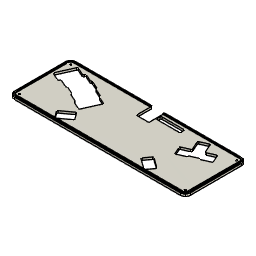
case-top v2 (Autodesk Fusion 360 design; units mm, degrees)
Autodesk Fusion 360 part; units mm, degrees
sketch "triplejump-brd" plane through (0, 0, 0) normal (0, 0, 1) x (1, 0, 0)
  line L0 (142.675, 106.5563) -> (142.925, 106.5563)
  line L1 (109.6125, 106.3063) -> (109.6125, 106.5563)
  line L2 (121.5187, 106.5563) -> (121.7687, 106.5563)
  line L3 (121.5187, 99.0562) -> (121.7687, 99.0562)
  line L4 (121.5187, 99.3062) -> (121.5187, 99.0562)
  line L5 (130.7687, 99.0562) -> (121.7687, 99.0562)
  line L6 (130.7687, 99.0562) -> (131.0187, 99.0562)
  line L7 (131.0187, 106.5563) -> (131.0187, 106.3063)
  line L8 (121.5187, 99.3062) -> (121.5187, 106.3063)
  line L9 (121.7687, 106.5563) -> (130.7687, 106.5563)
  line L10 (109.6125, 99.3062) -> (109.6125, 99.0562)
  line L11 (133.425, 99.0562) -> (133.675, 99.0562)
  line L12 (133.675, 106.5563) -> (142.675, 106.5563)
  line L13 (118.8625, 106.5563) -> (119.1125, 106.5563)
  line L14 (109.8625, 106.5563) -> (118.8625, 106.5563)
  line L15 (142.925, 99.0562) -> (142.925, 99.3062)
  line L16 (142.925, 106.3063) -> (142.925, 99.3062)
  line L17 (119.1125, 99.0562) -> (119.1125, 99.3062)
  line L18 (133.425, 106.5563) -> (133.675, 106.5563)
  line L19 (130.7687, 106.5563) -> (131.0187, 106.5563)
  line L20 (133.425, 99.3062) -> (133.425, 106.3063)
  line L21 (142.675, 99.0562) -> (142.925, 99.0562)
  line L22 (109.6125, 99.0562) -> (109.8625, 99.0562)
  spline S0 degree 3 poles (1.4645, 1.4645) (2.4021, 0.5268) (3.6739, 0) (5, 0) knots 0 0 0 0 1 1 1 1
  line L23 (133.425, 99.3062) -> (133.425, 99.0562)
  line L24 (133.425, 106.3063) -> (133.425, 106.5563)
  line L25 (142.925, 106.5563) -> (142.925, 106.3063)
  line L26 (121.5187, 106.3063) -> (121.5187, 106.5563)
  line L27 (118.8625, 99.0562) -> (109.8625, 99.0562)
  line L28 (119.1125, 106.5563) -> (119.1125, 106.3063)
  line L29 (142.675, 99.0562) -> (133.675, 99.0562)
  line L30 (119.1125, 106.3063) -> (119.1125, 99.3062)
  line L31 (118.8625, 99.0562) -> (119.1125, 99.0562)
  line L32 (109.6125, 106.5563) -> (109.8625, 106.5563)
  spline S1 degree 3 poles (335, 0) (336.3261, 0) (337.5979, 0.5268) (338.5355, 1.4645) knots 0 0 0 0 1 1 1 1
  line L33 (177, 112) -> (176.5, 112)
  line L34 (129.7687, 102.0563) -> (129.7687, 103.5563)
  line L35 (289.3678, 84.0164) -> (288.4543, 83.6096)
  line L36 (276.5782, 78.322) -> (276.1714, 79.2356)
  line L37 (110.8625, 103.5563) -> (110.8625, 102.0563)
  line L38 (271.7974, 91.5184) -> (270.8839, 91.1117)
  line L39 (54.537, 92.7011) -> (54.9437, 93.6146)
  line L40 (117.8625, 102.0563) -> (117.8625, 103.5563)
  line L41 (134.675, 103.5563) -> (134.675, 102.0563)
  line L42 (122.7687, 103.5563) -> (122.7687, 102.0563)
  spline S2 degree 3 poles (5, 112) (3.6739, 112) (2.4021, 111.4732) (1.4645, 110.5355) knots 0 0 0 0 1 1 1 1
  line L43 (131.0187, 99.0562) -> (131.0187, 99.3062)
  spline S3 degree 3 poles (0, 5) (0, 3.6739) (0.5268, 2.4021) (1.4645, 1.4645) knots 0 0 0 0 1 1 1 1
  line L44 (131.0187, 106.3063) -> (131.0187, 99.3062)
  line L45 (335, 112) -> (177, 112)
  spline S4 degree 3 poles (1.4645, 110.5355) (0.5268, 109.5979) (0, 108.3261) (0, 107) knots 0 0 0 0 1 1 1 1
  spline S5 degree 3 poles (338.5355, 1.4645) (339.4732, 2.4021) (340, 3.6739) (340, 5) knots 0 0 0 0 1 1 1 1
  line L46 (5, 0) -> (335, 0)
  line L47 (163, 112) -> (5, 112)
  line L48 (340, 5) -> (340, 107)
  spline S6 degree 3 poles (340, 107) (340, 108.3261) (339.4732, 109.5979) (338.5355, 110.5355) knots 0 0 0 0 1 1 1 1
  line L49 (0, 107) -> (0, 5)
  line L50 (163.5, 112) -> (163, 112)
  spline S7 degree 3 poles (338.5355, 110.5355) (337.5979, 111.4732) (336.3261, 112) (335, 112) knots 0 0 0 0 1 1 1 1
  line L51 (54.537, 92.7011) -> (55.4505, 92.2944)
  line L52 (288.9611, 84.9299) -> (289.3678, 84.0164)
  line L53 (140.425, 106.0563) -> (135.925, 106.0563)
  line L54 (283.6735, 96.806) -> (282.76, 96.3993)
  line L55 (59.8246, 104.5772) -> (60.2313, 105.4907)
  line L56 (73.021, 99.7964) -> (72.1074, 100.2032)
  line L57 (128.5187, 106.0563) -> (124.0187, 106.0563)
  line L58 (61.1449, 105.084) -> (60.2313, 105.4907)
  line L59 (283.6735, 96.806) -> (284.0802, 95.8925)
  line L60 (67.3266, 87.0068) -> (66.4131, 87.4135)
  line L61 (276.5782, 78.322) -> (277.4917, 78.7288)
  line L62 (112.1125, 99.5562) -> (116.6125, 99.5562)
  line L63 (66.4131, 87.4135) -> (67.3266, 87.0068)
  line L64 (288.4543, 83.6096) -> (289.3678, 84.0164)
  line L65 (67.7334, 87.9203) -> (67.3266, 87.0068)
  line L66 (141.675, 102.0563) -> (141.675, 103.5563)
  line L67 (124.0187, 99.5562) -> (128.5187, 99.5562)
  line L68 (116.6125, 106.0563) -> (112.1125, 106.0563)
  line L69 (135.925, 99.5562) -> (140.425, 99.5562)
  line L70 (73.021, 99.7964) -> (72.6142, 98.8829)
  line L71 (145.3312, 106.3063) -> (145.3312, 106.5563)
  line L72 (145.5812, 106.5563) -> (154.5812, 106.5563)
  line L73 (145.3312, 99.0562) -> (145.5812, 99.0562)
  line L74 (145.3312, 99.3062) -> (145.3312, 99.0562)
  line L75 (145.3312, 106.5563) -> (145.5812, 106.5563)
  line L76 (154.5812, 99.0562) -> (145.5812, 99.0562)
  line L77 (145.3312, 99.3062) -> (145.3312, 106.3063)
  line L78 (154.8312, 106.5563) -> (154.8312, 106.3063)
  line L79 (154.8312, 99.0562) -> (154.8312, 99.3062)
  line L80 (154.5812, 106.5563) -> (154.8312, 106.5563)
  line L81 (154.5812, 99.0562) -> (154.8312, 99.0562)
  line L82 (297.1161, 66.6133) -> (296.2026, 66.2066)
  line L83 (254.3169, 5.0503) -> (253.5079, 5.6381)
  line L84 (291.4218, 79.403) -> (290.5083, 78.9962)
  line L85 (88.7804, 24.6055) -> (87.9714, 24.0177)
  line L86 (88.7804, 24.6055) -> (89.3682, 23.7965)
  line L87 (85.6831, 5.0503) -> (86.4921, 5.6381)
  line L88 (254.8305, 80.332) -> (254.4237, 81.2455)
  line L89 (96.2004, 12.6915) -> (97.0094, 13.2793)
  line L90 (284.3265, 60.919) -> (285.2401, 61.3257)
  line L91 (260.118, 68.4559) -> (259.7113, 69.3694)
  line L92 (85.6831, 5.0503) -> (85.0953, 5.8593)
  line L93 (242.9906, 13.2793) -> (243.7996, 12.6915)
  line L94 (246.1187, 53.0628) -> (245.7119, 53.9763)
  line L95 (258.5016, 59.6706) -> (258.9083, 58.7571)
  line L96 (41.1761, 75.1935) -> (40.2625, 75.6002)
  line L97 (294.9241, 83.9526) -> (294.5174, 84.8661)
  line L98 (68.4801, 77.2672) -> (68.8868, 78.1808)
  line L99 (302.6725, 66.5495) -> (303.586, 66.9562)
  line L100 (296.2026, 66.2066) -> (297.1161, 66.6133)
  line L101 (254.9047, 5.8593) -> (254.3169, 5.0503)
  line L102 (267.2134, 86.9398) -> (267.6201, 86.0263)
  line L103 (326.5959, 94.0731) -> (327.0026, 93.1595)
  line L104 (63.1925, 65.3911) -> (63.5993, 66.3047)
  line L105 (297.8917, 79.7459) -> (296.9782, 79.3391)
  line L106 (250.6318, 23.7965) -> (251.2196, 24.6055)
  line L107 (267.2134, 86.9398) -> (266.2998, 86.5331)
  line L108 (253.5079, 5.6381) -> (254.3169, 5.0503)
  line L109 (296.7094, 67.5269) -> (297.1161, 66.6133)
  line L110 (262.5459, 16.3765) -> (261.9581, 15.5675)
  line L111 (279.5457, 74.1154) -> (278.6322, 73.7086)
  line L112 (260.118, 68.4559) -> (261.0316, 68.8626)
  line L113 (306.8002, 89.2401) -> (307.7138, 89.6469)
  line L114 (76.3889, 60.6104) -> (75.9822, 59.6968)
  line L115 (302.6725, 66.5495) -> (302.2657, 67.4631)
  line L116 (272.5009, 75.0637) -> (272.9077, 74.1502)
  line L117 (262.5459, 16.3765) -> (261.7368, 16.9643)
  line L118 (28.3864, 80.8878) -> (29.3, 80.4811)
  line L119 (334.751, 75.7565) -> (333.8374, 75.3498)
  line L120 (78.2632, 16.9643) -> (77.4541, 16.3765)
  line L121 (291.4218, 79.403) -> (291.8286, 78.4894)
  line L122 (242.9906, 13.2793) -> (243.5784, 14.0883)
  line L123 (75.0686, 60.1035) -> (75.9822, 59.6968)
  line L124 (321.3083, 105.9492) -> (320.3948, 105.5424)
  line L125 (251.4063, 41.1867) -> (252.3198, 41.5934)
  line L126 (252.0286, 24.0177) -> (251.2196, 24.6055)
  line L127 (333.8374, 75.3498) -> (334.751, 75.7565)
  line L128 (258.5016, 59.6706) -> (257.588, 59.2639)
  line L129 (284.3265, 60.919) -> (283.9198, 61.8326)
  line L130 (329.0567, 88.5461) -> (328.1431, 88.1394)
  line L131 (279.0389, 72.7951) -> (278.6322, 73.7086)
  line L132 (255.3373, 81.6523) -> (254.4237, 81.2455)
  line L133 (81.6765, 72.4864) -> (81.2697, 71.5729)
  line L134 (272.9077, 74.1502) -> (271.9941, 73.7435)
  line L135 (271.9941, 73.7435) -> (272.9077, 74.1502)
  line L136 (78.0419, 15.5675) -> (77.4541, 16.3765)
  line L137 (327.0026, 93.1595) -> (326.0891, 92.7528)
  line L138 (147.8312, 99.5562) -> (152.3312, 99.5562)
  line L139 (256.4476, 64.284) -> (255.534, 63.8773)
  line L140 (294.9241, 83.9526) -> (295.8377, 84.3593)
  line L141 (28.3864, 80.8878) -> (28.7932, 81.8013)
  line L142 (75.9822, 59.6968) -> (75.0686, 60.1035)
  line L143 (271.2906, 90.1981) -> (270.8839, 91.1117)
  line L144 (53.3659, 87.6977) -> (52.4523, 88.1045)
  line L145 (153.5812, 102.0563) -> (153.5812, 103.5563)
  line L146 (46.8704, 87.9831) -> (45.9568, 88.3899)
  line L147 (58.6341, 70.0273) -> (59.5477, 69.6205)
  line L148 (302.0195, 102.4365) -> (302.4262, 101.523)
  line L149 (40.2625, 75.6002) -> (41.1761, 75.1935)
  line L150 (96.4216, 14.0883) -> (97.0094, 13.2793)
  line L151 (316.6738, 81.9383) -> (316.267, 82.8518)
  line L152 (263.7892, 47.7945) -> (264.1959, 46.881)
  line L153 (326.0891, 92.7528) -> (327.0026, 93.1595)
  line L154 (52.0456, 87.1909) -> (52.4523, 88.1045)
  line L155 (81.6765, 72.4864) -> (80.7629, 72.8932)
  line L156 (309.7678, 85.0335) -> (308.8542, 84.6267)
  line L157 (263.2823, 46.4743) -> (264.1959, 46.881)
  line L158 (309.4322, 100.6616) -> (308.5187, 100.2549)
  line L159 (314.5486, 71.8371) -> (315.4621, 72.2438)
  line L160 (309.7678, 85.0335) -> (310.1745, 84.1199)
  line L161 (264.1959, 46.881) -> (263.2823, 46.4743)
  line L162 (321.9613, 70.0622) -> (322.8749, 70.4689)
  line L163 (34.9943, 93.2707) -> (34.0808, 93.6774)
  line L164 (302.0195, 102.4365) -> (301.1059, 102.0298)
  line L165 (307.7138, 89.6469) -> (306.8002, 89.2401)
  line L166 (46.8704, 87.9831) -> (46.4637, 87.0696)
  line L167 (297.3849, 78.4256) -> (296.9782, 79.3391)
  line L168 (290.1434, 97.1489) -> (289.2298, 96.7422)
  line L169 (33.674, 92.7639) -> (34.0808, 93.6774)
  line L170 (307.307, 90.5604) -> (307.7138, 89.6469)
  line L171 (314.213, 87.4652) -> (313.8063, 88.3788)
  line L172 (246.6255, 54.3831) -> (245.7119, 53.9763)
  line L173 (315.0554, 73.1574) -> (315.4621, 72.2438)
  line L174 (69.8004, 77.774) -> (68.8868, 78.1808)
  line L175 (251.4063, 41.1867) -> (250.9995, 42.1002)
  line L176 (46.758, 75.3148) -> (47.6716, 74.9081)
  line L177 (97.0094, 13.2793) -> (96.2004, 12.6915)
  line L178 (321.9613, 70.0622) -> (321.5546, 70.9757)
  line L179 (41.5828, 76.107) -> (41.1761, 75.1935)
  line L180 (238.8772, 71.7861) -> (237.9636, 71.3794)
  line L181 (280.656, 56.7472) -> (279.7425, 56.3404)
  line L182 (267.8664, 51.0528) -> (267.4596, 51.9664)
  line L183 (314.213, 87.4652) -> (315.1266, 87.872)
  line L184 (238.3703, 70.4658) -> (237.9636, 71.3794)
  line L185 (317.1806, 83.2586) -> (316.267, 82.8518)
  line L186 (263.0856, 64.2492) -> (262.1721, 63.8425)
  line L187 (334.3442, 76.67) -> (334.751, 75.7565)
  line L188 (274.9617, 69.5368) -> (275.3684, 68.6232)
  line L189 (315.4621, 72.2438) -> (314.5486, 71.8371)
  line L190 (267.8664, 51.0528) -> (268.7799, 51.4596)
  line L191 (329.0567, 88.5461) -> (329.4634, 87.6326)
  line L192 (63.1925, 65.3911) -> (64.1061, 64.9844)
  line L193 (255.534, 63.8773) -> (256.4476, 64.284)
  line L194 (250.7532, 77.0737) -> (251.16, 76.1601)
  line L195 (289.6366, 95.8286) -> (289.2298, 96.7422)
  line L196 (243.6579, 58.5897) -> (243.2512, 59.5033)
  line L197 (308.9254, 99.3413) -> (308.5187, 100.2549)
  line L198 (280.2493, 57.6607) -> (280.656, 56.7472)
  line L199 (321.3083, 105.9492) -> (321.7151, 105.0356)
  line L200 (250.7532, 77.0737) -> (249.8397, 76.6669)
  line L201 (65.242, 82.4102) -> (64.3284, 82.8169)
  line L202 (59.5477, 69.6205) -> (58.6341, 70.0273)
  line L203 (274.9617, 69.5368) -> (274.0482, 69.1301)
  line L204 (243.6579, 58.5897) -> (244.5715, 58.9965)
  line L205 (146.5812, 103.5563) -> (146.5812, 102.0563)
  line L206 (59.9544, 70.5341) -> (59.5477, 69.6205)
  line L207 (65.242, 82.4102) -> (64.8352, 81.4966)
  line L208 (46.758, 75.3148) -> (47.1648, 76.2284)
  line L209 (279.7425, 56.3404) -> (280.656, 56.7472)
  line L210 (152.3312, 106.0563) -> (147.8312, 106.0563)
  line L211 (262.5788, 62.9289) -> (262.1721, 63.8425)
  line L212 (256.0408, 65.1976) -> (256.4476, 64.284)
  circle A0 centre (5, 107) radius 1.6
  circle A1 centre (5, 5) radius 1.6
  circle A2 centre (335, 107) radius 1.6
  circle A3 centre (335, 5) radius 1.6
  spline S8 degree 3 poles (339.2426, 0.7574) (340.3676, 1.8823) (341, 3.4091) (341, 5) knots 0 0 0 0 1 1 1 1
  line L213 (341, 5) -> (341, 107)
  spline S9 degree 3 poles (341, 107) (341, 108.5909) (340.3676, 110.1177) (339.2426, 111.2426) knots 0 0 0 0 1 1 1 1
  spline S10 degree 3 poles (339.2426, 111.2426) (338.1177, 112.3676) (336.5909, 113) (335, 113) knots 0 0 0 0 1 1 1 1
  line L214 (335, 113) -> (177, 113)
  line L215 (177, 113) -> (5, 113)
  spline S11 degree 3 poles (5, 113) (3.4091, 113) (1.8823, 112.3676) (0.7574, 111.2426) knots 0 0 0 0 1 1 1 1
  spline S12 degree 3 poles (0.7574, 111.2426) (-0.3676, 110.1177) (-1, 108.5909) (-1, 107) knots 0 0 0 0 1 1 1 1
  line L216 (-1, 107) -> (-1, 5)
  spline S13 degree 3 poles (-1, 5) (-1, 3.4091) (-0.3676, 1.8823) (0.7574, 0.7574) knots 0 0 0 0 1 1 1 1
  spline S14 degree 3 poles (0.7574, 0.7574) (1.8823, -0.3676) (3.4091, -1) (5, -1) knots 0 0 0 0 1 1 1 1
  line L217 (5, -1) -> (335, -1)
  spline S15 degree 3 poles (335, -1) (336.5909, -1) (338.1177, -0.3676) (339.2426, 0.7574) knots 0 0 0 0 1 1 1 1
  line L218 (68.5336, 83.0202) -> (69.3276, 84.74)
  line L219 (75.6348, 98.9062) -> (69.3276, 84.74)
  line L220 (60.4613, 107.8512) -> (74.6212, 101.5468)
  line L221 (51.5191, 92.6839) -> (57.8207, 106.8376)
  line L222 (50.6964, 90.902) -> (51.5191, 92.6839)
  line L223 (34.3108, 96.038) -> (48.0671, 89.9133)
  line L224 (25.7725, 81.7779) -> (31.6702, 95.0243)
  line L225 (41.2587, 72.6938) -> (26.7862, 79.1374)
  line L226 (59.2192, 67.3038) -> (45.5688, 73.3814)
  line L227 (75.7522, 57.3363) -> (61.5922, 63.6407)
  line L228 (84.2904, 71.5963) -> (78.3927, 58.3499)
  line L229 (69.5359, 80.3547) -> (83.2768, 74.2369)
  line L230 (235.3496, 70.4892) -> (248.9957, 39.8398)
  line L231 (251.6363, 38.8261) -> (265.7962, 45.1306)
  line L232 (282.2563, 54.9968) -> (268.1688, 48.7246)
  line L233 (298.3054, 64.6799) -> (284.6289, 58.5908)
  line L234 (302.5639, 64.0382) -> (316.6513, 70.3103)
  line L235 (319.2919, 69.2967) -> (319.5508, 68.7153)
  line L236 (336.3513, 74.0061) -> (322.1913, 67.7016)
  line L237 (337.3649, 76.6466) -> (323.7189, 107.2961)
  line L238 (321.0783, 108.3097) -> (307.3295, 102.1883)
  line L239 (304.6889, 103.202) -> (304.43, 103.7834)
  line L240 (288.0406, 98.6757) -> (301.7895, 104.7971)
  line L241 (268.9449, 92.7114) -> (283.7822, 99.3173)
  line L242 (266.5723, 89.1173) -> (252.4847, 82.8451)
  line L243 (250.1121, 79.2512) -> (236.3633, 73.1298)
  line L244 (154.8312, 99.0562) -> (154.8312, 106.5563)
  line L245 (109.6125, 99.0562) -> (109.6125, 106.5563)
  line L246 (153.8312, 98.0562) -> (110.6125, 98.0562)
  line L247 (108.6125, 100.0562) -> (108.6125, 105.5563)
  line L248 (110.6125, 107.5563) -> (153.8312, 107.5563)
  line L249 (155.8312, 105.5563) -> (155.8312, 100.0562)
  line L250 (102.5792, 14.5449) -> (82.7583, 0.1441)
  line L251 (79.9647, 0.5866) -> (71.4418, 12.3173)
  line L252 (71.8843, 15.1109) -> (91.7052, 29.5117)
  line L253 (94.4988, 29.0692) -> (103.0217, 17.3385)
  line L254 (257.2417, 0.1441) -> (237.4208, 14.5449)
  line L255 (236.9783, 17.3385) -> (245.5012, 29.0692)
  line L256 (248.2948, 29.5117) -> (268.1157, 15.1109)
  line L257 (268.5582, 12.3173) -> (260.0353, 0.5866)
  arc A4 (60.4613, 107.8512) -> (57.8207, 106.8376) centre (59.6478, 106.0241) ccw
  arc A5 (75.6348, 98.9062) -> (74.6212, 101.5468) centre (73.8077, 99.7197) ccw
  arc A6 (68.5336, 83.0202) -> (69.5359, 80.3547) centre (70.3494, 82.1818) ccw
  arc A7 (84.2904, 71.5963) -> (83.2768, 74.2369) centre (82.4633, 72.4098) ccw
  arc A8 (75.7522, 57.3363) -> (78.3927, 58.3499) centre (76.5656, 59.1634) ccw
  arc A9 (60.4057, 65.4723) -> (61.5922, 63.6407) centre (62.4057, 65.4678) ccw
  arc A10 (60.4057, 65.4723) -> (59.2192, 67.3038) centre (58.4057, 65.4768) ccw
  arc A11 (45.5688, 73.3814) -> (43.4138, 73.0376) centre (44.7554, 71.5543) ccw
  arc A12 (41.2587, 72.6938) -> (43.4138, 73.0376) centre (42.0722, 74.5209) ccw
  arc A13 (25.7725, 81.7779) -> (26.7862, 79.1374) centre (27.5996, 80.9645) ccw
  arc A14 (34.3108, 96.038) -> (31.6702, 95.0243) centre (33.4973, 94.2109) ccw
  arc A15 (48.0671, 89.9133) -> (50.6964, 90.902) centre (48.8806, 91.7403) ccw
  arc A16 (94.4988, 29.0692) -> (91.7052, 29.5117) centre (92.8808, 27.8936) ccw
  arc A17 (102.5792, 14.5449) -> (103.0217, 17.3385) centre (101.4037, 16.1629) ccw
  arc A18 (79.9647, 0.5866) -> (82.7583, 0.1441) centre (81.5827, 1.7622) ccw
  arc A19 (71.8843, 15.1109) -> (71.4418, 12.3173) centre (73.0598, 13.4929) ccw
  arc A20 (248.2948, 29.5117) -> (245.5012, 29.0692) centre (247.1192, 27.8936) ccw
  arc A21 (268.5582, 12.3173) -> (268.1157, 15.1109) centre (266.9402, 13.4929) ccw
  arc A22 (257.2417, 0.1441) -> (260.0353, 0.5866) centre (258.4173, 1.7622) ccw
  arc A23 (236.9783, 17.3385) -> (237.4208, 14.5449) centre (238.5963, 16.1629) ccw
  arc A24 (236.3633, 73.1298) -> (235.3496, 70.4892) centre (237.1767, 71.3027) ccw
  arc A25 (248.9957, 39.8398) -> (251.6363, 38.8261) centre (250.8228, 40.6532) ccw
  arc A26 (265.7962, 45.1306) -> (266.9825, 46.9276) centre (264.9828, 46.9577) ccw
  arc A27 (268.1688, 48.7246) -> (266.9825, 46.9276) centre (268.9823, 46.8975) ccw
  arc A28 (282.2563, 54.9968) -> (283.4426, 56.7938) centre (281.4429, 56.8239) ccw
  arc A29 (284.6289, 58.5908) -> (283.4426, 56.7938) centre (285.4424, 56.7637) ccw
  arc A30 (300.4346, 64.359) -> (298.3054, 64.6799) centre (299.1188, 62.8528) ccw
  arc A31 (300.4346, 64.359) -> (302.5639, 64.0382) centre (301.7504, 65.8653) ccw
  arc A32 (319.2919, 69.2967) -> (316.6513, 70.3103) centre (317.4648, 68.4832) ccw
  arc A33 (319.5508, 68.7153) -> (322.1913, 67.7016) centre (321.3779, 69.5287) ccw
  arc A34 (336.3513, 74.0061) -> (337.3649, 76.6466) centre (335.5378, 75.8332) ccw
  arc A35 (323.7189, 107.2961) -> (321.0783, 108.3097) centre (321.8918, 106.4826) ccw
  arc A36 (304.6889, 103.202) -> (307.3295, 102.1883) centre (306.516, 104.0154) ccw
  arc A37 (304.43, 103.7834) -> (301.7895, 104.7971) centre (302.6029, 102.97) ccw
  arc A38 (285.9114, 98.9965) -> (288.0406, 98.6757) centre (287.2271, 100.5028) ccw
  arc A39 (285.9114, 98.9965) -> (283.7822, 99.3173) centre (284.5956, 97.4902) ccw
  arc A40 (266.5723, 89.1173) -> (267.7586, 90.9143) centre (265.7588, 90.9444) ccw
  arc A41 (268.9449, 92.7114) -> (267.7586, 90.9143) centre (269.7584, 90.8843) ccw
  arc A42 (250.1121, 79.2512) -> (251.2984, 81.0482) centre (249.2987, 81.0783) ccw
  arc A43 (252.4847, 82.8451) -> (251.2984, 81.0482) centre (253.2982, 81.0181) ccw
  line L258 (179, 112) -> (161, 112)
  line L259 (161, 112) -> (161, 88.5)
  line L260 (161, 88.5) -> (179, 88.5)
  line L261 (179, 88.5) -> (179, 112)
  line L262 (333.4123, 7.75) -> (331.8246, 5)
  line L263 (331.8246, 5) -> (333.4123, 2.25)
  line L264 (333.4123, 2.25) -> (336.5877, 2.25)
  line L265 (336.5877, 2.25) -> (338.1754, 5)
  line L266 (338.1754, 5) -> (336.5877, 7.75)
  line L267 (336.5877, 7.75) -> (333.4123, 7.75)
  line L268 (3.4123, 109.75) -> (1.8246, 107)
  line L269 (1.8246, 107) -> (3.4123, 104.25)
  line L270 (3.4123, 104.25) -> (6.5877, 104.25)
  line L271 (6.5877, 104.25) -> (8.1754, 107)
  line L272 (8.1754, 107) -> (6.5877, 109.75)
  line L273 (6.5877, 109.75) -> (3.4123, 109.75)
  line L274 (6.5877, 7.75) -> (3.4123, 7.75)
  line L275 (8.1754, 5) -> (6.5877, 7.75)
  line L276 (3.4123, 7.75) -> (1.8246, 5)
  line L277 (1.8246, 5) -> (3.4123, 2.25)
  line L278 (6.5877, 2.25) -> (8.1754, 5)
  line L279 (3.4123, 2.25) -> (6.5877, 2.25)
  line L280 (333.4123, 109.75) -> (331.8246, 107)
  line L281 (336.5877, 109.75) -> (333.4123, 109.75)
  line L282 (338.1754, 107) -> (336.5877, 109.75)
  line L283 (331.8246, 107) -> (333.4123, 104.25)
  line L284 (333.4123, 104.25) -> (336.5877, 104.25)
  line L285 (336.5877, 104.25) -> (338.1754, 107)
  arc A44 (77.9187, 97.8894) -> (75.6381, 103.8307) centre (73.8077, 99.7197) ccw
  line L286 (61.4781, 110.1351) -> (75.6381, 103.8307)
  arc A45 (61.4781, 110.1351) -> (55.5368, 107.8544) centre (59.6478, 106.0241) ccw
  line L287 (49.2421, 93.7163) -> (55.5368, 107.8544)
  line L288 (48.6333, 92.3977) -> (49.2421, 93.7163)
  line L289 (35.3276, 98.3218) -> (48.6333, 92.3977)
  arc A46 (35.3276, 98.3218) -> (29.3864, 96.0412) centre (33.4973, 94.2109) ccw
  line L290 (23.4887, 82.7948) -> (29.3864, 96.0412)
  arc A47 (23.4887, 82.7948) -> (25.7693, 76.8535) centre (27.5996, 80.9645) ccw
  line L291 (40.2419, 70.4099) -> (25.7693, 76.8535)
  arc A48 (40.2419, 70.4099) -> (44.8372, 70.9705) centre (42.0722, 74.5209) ccw
  line L292 (57.9171, 65.147) -> (44.8372, 70.9705)
  arc A49 (57.9171, 65.147) -> (60.5754, 61.3568) centre (62.4057, 65.4678) ccw
  line L293 (74.7353, 55.0524) -> (60.5754, 61.3568)
  arc A50 (74.7353, 55.0524) -> (80.6766, 57.3331) centre (76.5656, 59.1634) ccw
  line L294 (86.5743, 70.5795) -> (80.6766, 57.3331)
  arc A51 (86.5743, 70.5795) -> (84.2936, 76.5208) centre (82.4633, 72.4098) ccw
  line L295 (71.0158, 82.4324) -> (84.2936, 76.5208)
  line L296 (71.0158, 82.4324) -> (71.6046, 83.7076)
  line L297 (77.9187, 97.8894) -> (71.6046, 83.7076)
  arc A52 (108.6125, 100.0562) -> (110.6125, 98.0562) centre (110.6125, 100.0562) ccw
  arc A53 (110.6125, 107.5563) -> (108.6125, 105.5563) centre (110.6125, 105.5563) ccw
  arc A54 (155.8312, 105.5563) -> (153.8312, 107.5563) centre (153.8312, 105.5563) ccw
  arc A55 (153.8312, 98.0562) -> (155.8312, 100.0562) centre (153.8312, 100.0562) ccw
  spline S16 degree 3 poles (-0.6569, -0.6569) (0.8429, -2.1566) (2.8791, -3) (5, -3) knots 0 0 0 0 1 1 1 1
  line L298 (5, -3) -> (335, -3)
  spline S17 degree 3 poles (335, -3) (337.1209, -3) (339.1571, -2.1566) (340.6569, -0.6569) knots 0 0 0 0 1 1 1 1
  spline S18 degree 3 poles (340.6569, -0.6569) (342.1566, 0.8429) (343, 2.8791) (343, 5) knots 0 0 0 0 1 1 1 1
  line L299 (343, 5) -> (343, 107)
  spline S19 degree 3 poles (343, 107) (343, 109.1209) (342.1566, 111.1571) (340.6569, 112.6569) knots 0 0 0 0 1 1 1 1
  spline S20 degree 3 poles (340.6569, 112.6569) (339.1571, 114.1566) (337.1209, 115) (335, 115) knots 0 0 0 0 1 1 1 1
  line L300 (335, 115) -> (177, 115)
  line L301 (177, 115) -> (5, 115)
  spline S21 degree 3 poles (5, 115) (2.8791, 115) (0.8429, 114.1566) (-0.6569, 112.6569) knots 0 0 0 0 1 1 1 1
  spline S22 degree 3 poles (-0.6569, 112.6569) (-2.1566, 111.1571) (-3, 109.1209) (-3, 107) knots 0 0 0 0 1 1 1 1
  line L302 (-3, 107) -> (-3, 5)
  spline S23 degree 3 poles (-3, 5) (-3, 2.8791) (-2.1566, 0.8429) (-0.6569, -0.6569) knots 0 0 0 0 1 1 1 1
  spline S24 degree 3 poles (342.0711, 114.0711) (340.1966, 115.9456) (337.651, 117) (335, 117) knots 0 0 0 0 1 1 1 1
  line L303 (335, 117) -> (177, 117)
  line L304 (177, 117) -> (5, 117)
  spline S25 degree 3 poles (5, 117) (2.349, 117) (-0.1966, 115.9456) (-2.0711, 114.0711) knots 0 0 0 0 1 1 1 1
  spline S26 degree 3 poles (-2.0711, 114.0711) (-3.9456, 112.1966) (-5, 109.651) (-5, 107) knots 0 0 0 0 1 1 1 1
  line L305 (-5, 107) -> (-5, 5)
  spline S27 degree 3 poles (-5, 5) (-5, 2.349) (-3.9456, -0.1966) (-2.0711, -2.0711) knots 0 0 0 0 1 1 1 1
  spline S28 degree 3 poles (-2.0711, -2.0711) (-0.1966, -3.9456) (2.349, -5) (5, -5) knots 0 0 0 0 1 1 1 1
  line L306 (5, -5) -> (335, -5)
  spline S29 degree 3 poles (335, -5) (337.651, -5) (340.1966, -3.9456) (342.0711, -2.0711) knots 0 0 0 0 1 1 1 1
  spline S30 degree 3 poles (342.0711, -2.0711) (343.9456, -0.1966) (345, 2.349) (345, 5) knots 0 0 0 0 1 1 1 1
  line L307 (345, 5) -> (345, 107)
  spline S31 degree 3 poles (345, 107) (345, 109.651) (343.9456, 112.1966) (342.0711, 114.0711) knots 0 0 0 0 1 1 1 1
  arc A56 (158.3312, 105.5563) -> (153.8312, 110.0563) centre (153.8312, 105.5563) ccw
  line L308 (110.6125, 110.0563) -> (153.8312, 110.0563)
  arc A57 (110.6125, 110.0563) -> (106.1125, 105.5563) centre (110.6125, 105.5563) ccw
  line L309 (106.1125, 100.0562) -> (106.1125, 105.5563)
  arc A58 (106.1125, 100.0562) -> (110.6125, 95.5562) centre (110.6125, 100.0562) ccw
  line L310 (153.8312, 95.5562) -> (110.6125, 95.5562)
  arc A59 (153.8312, 95.5562) -> (158.3312, 100.0562) centre (153.8312, 100.0562) ccw
  line L311 (158.3312, 105.5563) -> (158.3312, 100.0562)
  arc A60 (96.5213, 30.5387) -> (90.2357, 31.5342) centre (92.8808, 27.8936) ccw
  line L312 (70.4148, 17.1335) -> (90.2357, 31.5342)
  arc A61 (70.4148, 17.1335) -> (69.4193, 10.8479) centre (73.0598, 13.4929) ccw
  line L313 (77.9422, -0.8829) -> (69.4193, 10.8479)
  arc A62 (77.9422, -0.8829) -> (84.2278, -1.8784) centre (81.5827, 1.7622) ccw
  line L314 (104.0487, 12.5223) -> (84.2278, -1.8784)
  arc A63 (104.0487, 12.5223) -> (105.0442, 18.8079) centre (101.4037, 16.1629) ccw
  line L315 (96.5213, 30.5387) -> (105.0442, 18.8079)
  arc A64 (270.5807, 10.8479) -> (269.5852, 17.1335) centre (266.9402, 13.4929) ccw
  line L316 (249.7643, 31.5342) -> (269.5852, 17.1335)
  arc A65 (249.7643, 31.5342) -> (243.4787, 30.5387) centre (247.1192, 27.8936) ccw
  line L317 (234.9558, 18.8079) -> (243.4787, 30.5387)
  arc A66 (234.9558, 18.8079) -> (235.9513, 12.5223) centre (238.5963, 16.1629) ccw
  line L318 (255.7722, -1.8784) -> (235.9513, 12.5223)
  arc A67 (255.7722, -1.8784) -> (262.0578, -0.8829) centre (258.4173, 1.7622) ccw
  line L319 (270.5807, 10.8479) -> (262.0578, -0.8829)
  arc A68 (283.2732, 52.7129) -> (285.9257, 56.4315) centre (281.4429, 56.8239) ccw
  line L320 (299.0422, 62.2714) -> (285.9257, 56.4315)
  arc A69 (299.0422, 62.2714) -> (303.5807, 61.7543) centre (301.7504, 65.8653) ccw
  line L321 (303.5807, 61.7543) -> (317.2114, 67.8231)
  line L322 (317.2114, 67.8231) -> (317.2669, 67.6984)
  arc A70 (317.2669, 67.6984) -> (323.2082, 65.4178) centre (321.3779, 69.5287) ccw
  line L323 (337.3681, 71.7222) -> (323.2082, 65.4178)
  arc A71 (337.3681, 71.7222) -> (339.6488, 77.6635) centre (335.5378, 75.8332) ccw
  line L324 (339.6488, 77.6635) -> (326.0027, 108.3129)
  arc A72 (326.0027, 108.3129) -> (320.0615, 110.5936) centre (321.8918, 106.4826) ccw
  line L325 (320.0615, 110.5936) -> (306.7694, 104.6756)
  line L326 (306.7694, 104.6756) -> (306.7139, 104.8003)
  arc A73 (306.7139, 104.8003) -> (300.7726, 107.0809) centre (302.6029, 102.97) ccw
  line L327 (287.3037, 101.0842) -> (300.7726, 107.0809)
  arc A74 (287.3037, 101.0842) -> (282.7653, 101.6012) centre (284.5956, 97.4902) ccw
  line L328 (267.9281, 94.9952) -> (282.7653, 101.6012)
  arc A75 (267.9281, 94.9952) -> (265.2755, 91.2766) centre (269.7584, 90.8843) ccw
  line L329 (265.2755, 91.2766) -> (251.4679, 85.129)
  arc A76 (251.4679, 85.129) -> (248.8153, 81.4104) centre (253.2982, 81.0181) ccw
  line L330 (248.8153, 81.4104) -> (235.3464, 75.4137)
  arc A77 (235.3464, 75.4137) -> (233.0658, 69.4724) centre (237.1767, 71.3027) ccw
  line L331 (233.0658, 69.4724) -> (246.7119, 38.8229)
  arc A78 (246.7119, 38.8229) -> (252.6531, 36.5423) centre (250.8228, 40.6532) ccw
  line L332 (252.6531, 36.5423) -> (266.8131, 42.8467)
  arc A79 (266.8131, 42.8467) -> (269.4656, 46.5654) centre (264.9828, 46.9577) ccw
  line L333 (283.2732, 52.7129) -> (269.4656, 46.5654)
  line L334 (161, 112) -> (179, 112)
  line L335 (179, 112) -> (179, 117)
  line L336 (179, 117) -> (161, 117)
  line L337 (161, 117) -> (161, 112)
  line L338 (161, 117) -> (161, 88.5)
  line L339 (179, 88.5) -> (179, 117)
  line L340 (157.5, 115) -> (157.5, 87)
  line L341 (159.5, 85) -> (180.5, 85)
  line L342 (182.5, 87) -> (182.5, 115)
  line L343 (5, 117) -> (155.5, 117)
  line L344 (184.5, 117) -> (335, 117)
  arc A80 (157.5, 87) -> (159.5, 85) centre (159.5, 87) ccw
  arc A81 (180.5, 85) -> (182.5, 87) centre (180.5, 87) ccw
  arc A82 (184.5, 117) -> (182.5, 115) centre (184.5, 115) ccw
  arc A83 (157.5, 115) -> (155.5, 117) centre (155.5, 115) ccw
  circle A84 centre (5, 107) radius 3
  circle A85 centre (5, 5) radius 3
  circle A86 centre (335, 5) radius 3
  circle A87 centre (335, 107) radius 3
  point P0 (335, 5)
  point P1 (335, 5)
  dimension "d25" = 2
  dimension "d28" = -2.5
  dimension "d29" = 2
  dimension "d30" = 2
  dimension "d31" = 2
  dimension "d32" = 2
  dimension "d33" = 4
  dimension "d34" = -2.5
  dimension "d35" = -2.5
  dimension "d36" = -2.5
  dimension "d37" = -2.5
  dimension "d60" = 2
  dimension "d61" = 2
  dimension "d62" = 2
  dimension "d63" = 2
  constraint perpendicular L80 L244
  constraint perpendicular L32 L245
  constraint tangent L220 A4
  constraint tangent L221 A4
  constraint tangent L219 A5
  constraint tangent L220 A5
  constraint equal A4 A5
  constraint tangent L218 A6
  constraint tangent L229 A6
  constraint equal A4 A6
  constraint tangent L229 A7
  constraint tangent L228 A7
  constraint equal A4 A7
  constraint tangent L228 A8
  constraint tangent L227 A8
  constraint equal A4 A8
  constraint tangent L227 A9
  constraint equal A4 A9
  constraint tangent L226 A10
  constraint tangent A9 A10
  constraint equal A4 A10
  constraint tangent L226 A11
  constraint equal A4 A11
  constraint tangent L225 A12
  constraint tangent A11 A12
  constraint equal A4 A12
  constraint tangent L225 A13
  constraint tangent L224 A13
  constraint equal A4 A13
  constraint tangent L224 A14
  constraint tangent L223 A14
  constraint equal A4 A14
  constraint tangent L223 A15
  constraint tangent L222 A15
  constraint equal A4 A15
  constraint tangent L252 A16
  constraint tangent L253 A16
  constraint equal A4 A16
  constraint tangent L253 A17
  constraint tangent L250 A17
  constraint equal A4 A17
  constraint tangent L250 A18
  constraint tangent L251 A18
  constraint equal A4 A18
  constraint tangent L251 A19
  constraint tangent L252 A19
  constraint equal A4 A19
  constraint tangent L255 A20
  constraint tangent L256 A20
  constraint equal A4 A20
  constraint tangent L257 A21
  constraint tangent L256 A21
  constraint equal A4 A21
  constraint tangent L257 A22
  constraint tangent L254 A22
  constraint equal A4 A22
  constraint tangent L254 A23
  constraint tangent L255 A23
  constraint equal A4 A23
  constraint tangent L243 A24
  constraint tangent L230 A24
  constraint equal A4 A24
  constraint tangent L230 A25
  constraint tangent L231 A25
  constraint equal A4 A25
  constraint tangent L231 A26
  constraint equal A4 A26
  constraint tangent L232 A27
  constraint tangent A26 A27
  constraint equal A4 A27
  constraint tangent L232 A28
  constraint equal A4 A28
  constraint tangent L233 A29
  constraint tangent A28 A29
  constraint equal A4 A29
  constraint tangent L233 A30
  constraint equal A4 A30
  constraint tangent L234 A31
  constraint tangent A30 A31
  constraint equal A4 A31
  constraint tangent L234 A32
  constraint tangent L235 A32
  constraint equal A4 A32
  constraint tangent L235 A33
  constraint tangent L236 A33
  constraint equal A4 A33
  constraint tangent L236 A34
  constraint tangent L237 A34
  constraint equal A4 A34
  constraint tangent L237 A35
  constraint tangent L238 A35
  constraint equal A4 A35
  constraint tangent L238 A36
  constraint tangent L239 A36
  constraint equal A4 A36
  constraint tangent L239 A37
  constraint tangent L240 A37
  constraint equal A4 A37
  constraint tangent L240 A38
  constraint equal A4 A38
  constraint tangent L241 A39
  constraint tangent A38 A39
  constraint equal A4 A39
  constraint tangent L242 A40
  constraint equal A4 A40
  constraint tangent L241 A41
  constraint tangent A40 A41
  constraint equal A4 A41
  constraint tangent L243 A42
  constraint equal A4 A42
  constraint tangent L242 A43
  constraint tangent A42 A43
  constraint equal A4 A43
  constraint horizontal L258
  constraint vertical L259
  constraint horizontal L260
  constraint vertical L261
  constraint coincident P1 P0
  constraint tangent L246 A52
  constraint tangent L248 A53
  constraint tangent L247 A53
  constraint tangent L248 A54
  constraint tangent L249 A54
  constraint equal A53 A54
  constraint tangent L249 A55
  constraint tangent L246 A55
  constraint horizontal L334
  constraint vertical L335
  constraint horizontal L336
  constraint vertical L337
  constraint coincident L303 L335.end
  constraint perpendicular L336 L339
  constraint tangent L340 A80
  constraint tangent L341 A80
  constraint tangent L341 A81
  constraint tangent L342 A81
  constraint tangent L344 A82
  constraint tangent L342 A82
  constraint tangent L340 A83
  constraint tangent L343 A83
  constraint concentric A0 A84
  constraint concentric A1 A85
  constraint concentric A2 A87
  measures "d25" radius of A4
  measures "d29" radius of A52
  measures "d30" radius of A53
  measures "d31" radius of A55
  measures "d60" radius of A80
  measures "d61" radius of A81
  measures "d62" radius of A82
  measures "d63" radius of A83
extrude "Extrude12" add sketch "triplejump-brd" along normal blind 1.6 from surface at 4.2 contours S8 L213 S9 S10 L214 L215 S11 S12 L216 S13 S14 L217 S15 S16 L298 S17 S18 L299 S19 S20 L300 L301 S21 S22 L302 S23 A62 L314 L318 A67 L340 L342 | L217 A62 L314 | L217 L318 A67 makes body 1
extrude "Extrude13" add sketch "triplejump-brd" along normal blind 4.2 from surface at 5.8 separate body contours S0 S1 S2 S3 L45 S4 S5 L46 L47 L48 S6 L49 S7 A56 L308 A57 L309 A58 L310 A59 A60 L312 A61 L313 L314 A63 L315 A64 L316 A65 L317 A66 L318 L319 A68 L320 A69 L321 L322 A70 L323 A71 L324 A72 L325 L326 A73 L327 A74 L328 A75 L329 A76 L330 A77 L331 A78 L332 A79 L333 L340 L341 L342 A80 A81 | S0 S2 S3 S4 L46 L47 L49 L215 S11 S12 L216 S13 S14 L217 L313 A62 L340 | L46 L250 L251 L252 L253 A16 A17 A18 A19 A60 L312 A61 L313 L314 A63 L315 | L46 L217 A18 L313 A62 L314 | S8 L213 S9 S10 L214 L215 S11 S12 L216 S13 S14 L217 S15 S16 L298 S17 S18 L299 S19 S20 L300 L301 S21 S22 L302 S23 A62 L314 L318 A67 L340 L342 | L217 A62 L314 | L46 L217 L314 L318 | L46 L254 L255 L256 L257 A20 A21 A22 A23 A64 L316 A65 L317 A66 L318 L319 | L46 L217 A22 L318 A67 L319 | L217 L318 A67 | A56 L308 A57 L309 A58 L310 A59 L340 | S1 L45 S5 L46 L48 S6 S7 S8 L213 S9 S10 L214 L217 S15 A67 L319 A71 L342 | S16 L298 S17 S18 L299 S19 S20 L300 L301 S21 S22 L302 S23 S24 L303 L304 S25 S26 L305 S27 S28 L306 S29 S30 L307 S31 L343 L344 A82 A83 | L48 A68 L320 A69 L321 L322 A70 L323 A71 L324 A72 L325 L326 A73 L327 A74 L328 A75 L329 A76 L330 A77 L331 A78 L332 A79 L333 | L48 A71 | L262 L267 A86 | L262 L263 L264 L265 L266 L267 A86 | L262 A86 | L267 A86 | L262 L263 A86 | L266 L267 A86 | L263 A86 | L266 A86 | L263 L264 A86 | L265 L266 A86 | L264 A86 | L264 L265 A86 | L265 A86 | L268 L273 A84 | L268 L269 L270 L271 L272 L273 A84 | L268 A84 | L273 A84 | L268 L269 A84 | L272 L273 A84 | L269 A84 | L272 A84 | L269 L270 A84 | L271 L272 A84 | L270 A84 | L270 L271 A84 | L271 A84 | L274 L275 A85 | L274 L275 L276 L277 L278 L279 A85 | L274 A85 | L275 A85 | L274 L276 A85 | L275 L278 A85 | L276 A85 | L276 L277 A85 | L278 A85 | L277 A85 | L278 L279 A85 | L277 L279 A85 | L279 A85 | L280 L281 A87 | L280 L281 L282 L283 L284 L285 A87 | L280 A87 | L281 A87 | L280 L283 A87 | L281 L282 A87 | L283 A87 | L282 A87 | L283 L284 A87 | L282 L285 A87 | L284 A87 | L284 L285 A87 | L285 A87 | A44 L286 A45 L287 L288 L289 A46 L290 A47 L291 A48 L292 A49 L293 A50 L294 A51 L295 L296 L297 makes body 2
chamfer "Chamfer1" distance 1.4 distance2 2 1 edges at (3.5083, 107.5786, 10) measured on face at (166.5, 39.1086, 10) on bodies 2
chamfer "Chamfer2" distance 1.4 distance2 2 1 edges at (3.5083, 5.5786, 10) measured on face at (166.5, 39.1086, 10) on bodies 2
chamfer "Chamfer3" distance 1.4 distance2 2 1 edges at (333.5083, 5.5786, 10) measured on face at (166.5, 39.1086, 10) on bodies 2
chamfer "Chamfer4" distance 1.4 distance2 2 1 edges at (333.5083, 107.5786, 10) measured on face at (166.5, 39.1086, 10) on bodies 2
move_body "Move1" bodies 2 1 to x (-1, 0, 0) y (0, 1, 0) z (0, 0, -1) at (-10.0001, 0, 11.5999)
move_body "Move2" bodies 2 1 to x (1, 0, 0) y (0, 1, 0) z (0, 0, 1) at (0, 0, -1.6)
extrude "Extrude1" [suppressed]
ref_plane "WorkPlane1" through (170, 56, 0.8) normal (0, 0, 1) x (1, 0, 0)
extrude "Extrude2" [suppressed]
ref_plane "WorkPlane2" through (170, 56, 4) normal (0, 0, 1) x (1, 0, 0)
extrude "Extrude3" [suppressed]
ref_plane "WorkPlane3" through (170, 56, 6.5) normal (0, 0, 1) x (1, 0, 0)
extrude "Extrude4" [suppressed]
extrude "Extrude5" [suppressed]
named bodies: "PCB", "t1.6", "t4.2"
